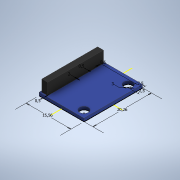
# Autodesk Inventor part: Gyrosensor
Saved by Autodesk Inventor 2021 (Build 250183000, 183)
## iProperties
Created: 2020-12-16
Part Number: Gyrosensor
Material: Generisch
Document SubType Name: Modeling
Designer: laure
Density: 1 g/cm^3
Appearance: Vorgabe
Author: laure
Autodesk Inventor part; units mm, degrees
ref_plane "YZ Plane" through (0, 0, 0) normal (1, 0, 0) x (0, 1, 0)
ref_plane "XZ Plane" through (0, 0, 0) normal (0, 1, 0) x (-1, 0, 0)
ref_plane "XY Plane" through (0, 0, 0) normal (0, 0, 1) x (1, 0, 0)
sketch "Skizze1" plane through (0, 0, 0) normal (0, 1, 0) x (-1, 0, 0)
  line L0 (-7.78, -10.13) -> (7.78, -10.13)
  line L1 (7.78, -10.13) -> (7.78, 10.13)
  line L2 (7.78, 10.13) -> (-7.78, 10.13)
  line L3 (-7.78, 10.13) -> (-7.78, -10.13)
  line L4 (0, -14.182) -> (0, 14.182) projected
  line L5 (10.892, 0) -> (-10.892, 0) projected
  circle A0 centre (-5.28, -7.63) radius 1.5
  circle A1 centre (-5.28, 7.63) radius 1.5
  line L6 (7.28, -9.63) -> (5.28, -9.63)
  line L7 (5.28, -9.63) -> (5.28, 9.63)
  line L8 (5.28, 9.63) -> (7.28, 9.63)
  line L9 (7.28, 9.63) -> (7.28, -9.63)
  point P0 (0, 0)
  dimension "d0" = 15.56
  dimension "d1" = 20.26
  dimension "d2" = 3
  dimension "d3" = 2.5
  dimension "d4" = 2.5
  dimension "d5" = 0.5
  dimension "d6" = 0.5
  dimension "d7" = 0.5
  dimension "d8" = 2
  constraints: 16 end point, 4 parallel, 2 centre point, 2 horizontal, 2 perpendicular, 1 symmetric about line, 3 other
  measures "d0" distance of L1.end L2.end
  measures "d1" distance of L0.end L1.end
  measures "d2" diameter of A0
  measures "d3" distance from line of L0 A0.centre
  measures "d4" distance from line of L3 A0.centre
  measures "d5" distance between parallel lines of L9 L1
  measures "d6" distance between parallel lines of L0 L6
  measures "d7" distance between parallel lines of L8 L2
  measures "d8" distance between parallel lines of L7 L9
extrude "Extrusion1" add sketch "Skizze1" along normal blind 1
extrude "Extrusion2" add sketch "Skizze1" along normal blind 5 contours L7 L8 L9 L5 | L5 L9 L6 L7
